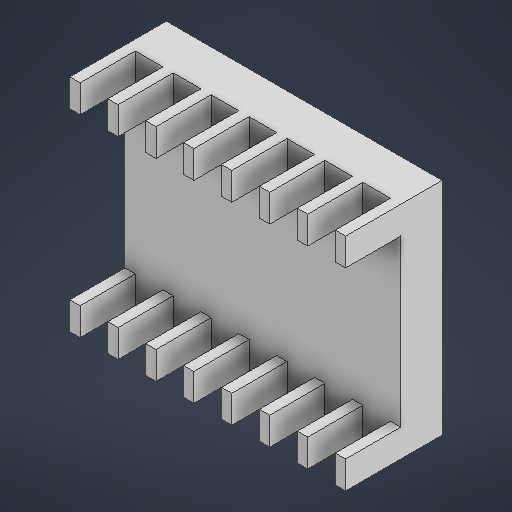
# Autodesk Inventor part: driver DRV8825
Saved by Autodesk Inventor 2026.2 (Build 302298010, 298A)
## iProperties
Created: 2026-03-17
Part Number: driver DRV8825
Material: Générique
Document SubType Name: Modeling
Designer: cleml
Density: 1 g/cm^3
Appearance: Par défaut
Author: cleml
Autodesk Inventor part; units mm, degrees
ref_plane "YZ Plane" through (0, 0, 0) normal (1, 0, 0) x (0, 1, 0)
ref_plane "XZ Plane" through (0, 0, 0) normal (0, 1, 0) x (-1, 0, 0)
ref_plane "XY Plane" through (0, 0, 0) normal (0, 0, 1) x (1, 0, 0)
sketch "Esquisse1" plane through (0, 0, 0) normal (0, 0, 1) x (1, 0, 0)
  line L0 (0, 0) -> (20, 0)
  line L1 (20, 0) -> (20, 16)
  line L2 (20, 16) -> (0, 16)
  line L3 (0, 16) -> (0, 0)
  dimension "d0" = 20
  dimension "d1" = 16
  constraints: 8 end point, 2 parallel, 1 horizontal, 1 perpendicular
  measures "d0" distance of L1.end L2.end
  measures "d1" distance of L0.end L1.end
extrude "Extrusion1" add sketch "Esquisse1" along normal blind 3
sketch "Esquisse2" plane through (0, 0, 3) normal (0, 0, 1) x (1, 0, 0)
  line L0 (20, 0) -> (20, 16) projected
  line L1 (20, 8) -> (0, 8)
  line L2 (0, 16) -> (0, 0) projected
  line L3 (20, 16) -> (0, 16)
  line L4 (0, 16) -> (0, 14)
  line L5 (0, 14) -> (20, 14)
  line L6 (20, 14) -> (20, 16)
  line L7 (20, 16) -> (19.25, 16)
  line L8 (19.25, 16) -> (19.25, 14)
  line L9 (19.25, 14) -> (20, 14)
  line L10 (20, 14) -> (20, 16)
  line L11 (19.25, 14) -> (17.25, 14)
  line L12 (17.25, 14) -> (17.25, 16)
  line L13 (17.25, 16) -> (16.5, 16)
  line L14 (16.5, 16) -> (16.5, 14)
  line L15 (16.5, 14) -> (17.25, 14)
  line L16 (17.25, 14) -> (17.25, 16)
  line L17 (16.5, 14) -> (14.5, 14)
  line L18 (14.5, 14) -> (14.5, 16)
  line L19 (14.5, 16) -> (13.75, 16)
  line L20 (13.75, 16) -> (13.75, 14)
  line L21 (13.75, 14) -> (14.5, 14)
  line L22 (14.5, 14) -> (14.5, 16)
  line L23 (13.75, 14) -> (11.75, 14)
  line L24 (11.75, 14) -> (11.75, 16)
  line L25 (11.75, 16) -> (11, 16)
  line L26 (11, 16) -> (11, 14)
  line L27 (11, 14) -> (11.75, 14)
  line L28 (11.75, 14) -> (11.75, 16)
  line L29 (11, 14) -> (9, 14)
  line L30 (9, 14) -> (9, 16)
  line L31 (9, 16) -> (8.25, 16)
  line L32 (8.25, 16) -> (8.25, 14)
  line L33 (8.25, 14) -> (9, 14)
  line L34 (9, 14) -> (9, 16)
  line L35 (8.25, 14) -> (6.25, 14)
  line L36 (6.25, 14) -> (6.25, 16)
  line L37 (6.25, 16) -> (5.5, 16)
  line L38 (5.5, 16) -> (5.5, 14)
  line L39 (5.5, 14) -> (6.25, 14)
  line L40 (6.25, 14) -> (6.25, 16)
  line L41 (5.5, 14) -> (3.5, 14)
  line L42 (3.5, 14) -> (3.5, 16)
  line L43 (3.5, 16) -> (2.75, 16)
  line L44 (2.75, 16) -> (2.75, 14)
  line L45 (2.75, 14) -> (3.5, 14)
  line L46 (3.5, 14) -> (3.5, 16)
  line L47 (2.75, 14) -> (0.75, 14)
  line L48 (0.75, 14) -> (0.75, 16)
  line L49 (20, 0) -> (0, 0)
  line L50 (0, 0) -> (0, 2)
  line L51 (0, 2) -> (20, 2)
  line L52 (20, 2) -> (20, 0)
  line L53 (20, 0) -> (19.25, 0)
  line L54 (19.25, 0) -> (19.25, 2)
  line L55 (19.25, 2) -> (20, 2)
  line L56 (20, 2) -> (20, 0)
  line L57 (19.25, 2) -> (17.25, 2)
  line L58 (17.25, 2) -> (17.25, 0)
  line L59 (17.25, 0) -> (16.5, 0)
  line L60 (16.5, 0) -> (16.5, 2)
  line L61 (16.5, 2) -> (17.25, 2)
  line L62 (17.25, 2) -> (17.25, 0)
  line L63 (16.5, 2) -> (14.5, 2)
  line L64 (14.5, 2) -> (14.5, 0)
  line L65 (14.5, 0) -> (13.75, 0)
  line L66 (13.75, 0) -> (13.75, 2)
  line L67 (13.75, 2) -> (14.5, 2)
  line L68 (14.5, 2) -> (14.5, 0)
  line L69 (13.75, 2) -> (11.75, 2)
  line L70 (11.75, 2) -> (11.75, 0)
  line L71 (11.75, 0) -> (11, 0)
  line L72 (11, 0) -> (11, 2)
  line L73 (11, 2) -> (11.75, 2)
  line L74 (11.75, 2) -> (11.75, 0)
  line L75 (11, 2) -> (9, 2)
  line L76 (9, 2) -> (9, 0)
  line L77 (9, 0) -> (8.25, 0)
  line L78 (8.25, 0) -> (8.25, 2)
  line L79 (8.25, 2) -> (9, 2)
  line L80 (9, 2) -> (9, 0)
  line L81 (8.25, 2) -> (6.25, 2)
  line L82 (6.25, 2) -> (6.25, 0)
  line L83 (6.25, 0) -> (5.5, 0)
  line L84 (5.5, 0) -> (5.5, 2)
  line L85 (5.5, 2) -> (6.25, 2)
  line L86 (6.25, 2) -> (6.25, 0)
  line L87 (5.5, 2) -> (3.5, 2)
  line L88 (3.5, 2) -> (3.5, 0)
  line L89 (3.5, 0) -> (2.75, 0)
  line L90 (2.75, 0) -> (2.75, 2)
  line L91 (2.75, 2) -> (3.5, 2)
  line L92 (3.5, 2) -> (3.5, 0)
  line L93 (2.75, 2) -> (0.75, 2)
  line L94 (0.75, 2) -> (0.75, 0)
  point P0 (0, 0)
  dimension "d4" = 2
  dimension "d5" = 0.75
  dimension "d6" = 2
  dimension "d7" = 2
  dimension "d8" = 2
  dimension "d9" = 2
  dimension "d10" = 2
  dimension "d11" = 2
  dimension "d12" = 2
  constraints: 186 end point, 45 symmetric about line, 16 parallel, 8 horizontal, 8 perpendicular, 7 point on line, 2 midpoint, 1 vertical
  measures "d4" distance between parallel lines of L3 L5
  measures "d5" distance between parallel lines of L0 L8
  measures "d6" distance of L8.end L11.end
  measures "d7" distance of L14.end L17.end
  measures "d8" distance of L20.end L23.end
  measures "d9" distance of L26.end L29.end
  measures "d10" distance of L32.end L35.end
  measures "d11" distance of L38.end L41.end
  measures "d12" distance of L44.end L47.end
extrude "Extrusion2" add sketch "Esquisse2" along normal blind 4 contours L49 L54 L51 L0 | L49 L60 L51 L58 | L5 L8 L3 L0 | L2 L3 L48 L5 | L51 L94 L49 L2 | L49 L66 L51 L64 | L5 L14 L3 L12 | L44 L3 L42 L5 | L51 L88 L49 L90 | L49 L72 L51 L70 | L5 L20 L3 L18 | L38 L3 L36 L5 | L51 L82 L49 L84 | L49 L78 L51 L76 | L5 L26 L3 L24 | L32 L3 L30 L5
